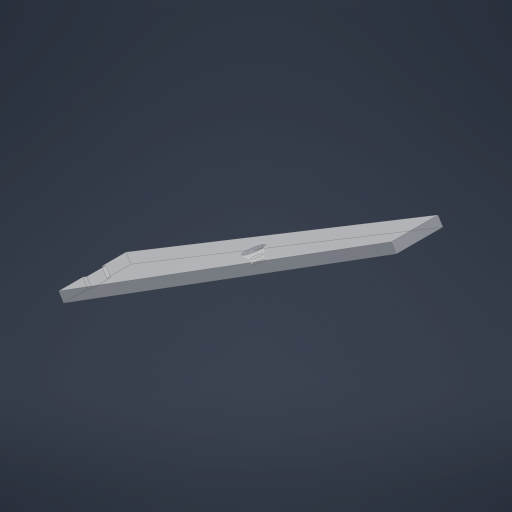
# Autodesk Inventor part: Touch Fifth
Saved by Autodesk Inventor 2023 (Build 270158000, 158)
## iProperties
Created: 2022-06-12
Part Number: Touch Fifth
Material: Polycarbonate, Clear
Document SubType Name: Modeling
Designer: FizzyApple12
Density: 1.2 g/cm^3
Appearance: Polycarbonate - Clear
Author: FizzyApple12
Autodesk Inventor part; units mm, degrees
ref_plane "XZ Plane" through (0, 0, 0) normal (0, 1, 0) x (-1, 0, 0)
sketch "Sketch1" plane through (0, 0, 0) normal (1, 0, 0) x (0, 1, 0)
  circle A0 centre (0, 0) radius 431.8 construction
  line L0 (-431.2082, -22.5987) -> (-431.2082, 22.5987)
  line L1 (-431.2082, -22.5987) -> (-386.0109, -22.5987) construction
  line L2 (-431.2082, -22.5987) -> (0, 0) construction
  line L3 (0, 0) -> (-431.2082, 22.5987) construction
  dimension "d0" = 863.6
  dimension "d3" = 90
  dimension "d4" = 6
  constraints: 8 end point, 2 point on circle, 1 centre point, 1 coincident, 1 horizontal, 1 perpendicular
  measures "d0" diameter of A0
  measures "d3" angle of L1 L0
  measures "d4" angle of L3 L2
ref_plane "Work Plane1" through (216.1794, 0, 0) normal (1, 0, 0) x (0, 1, 0)
sketch "Sketch2" plane through (216.1794, 0, 0) normal (1, 0, 0) x (0, 1, 0)
  circle A0 centre (0, 0) radius 298.45 construction
  line L0 (-298.041, 15.6197) -> (-298.041, -15.6197)
  line L1 (-298.041, 15.6197) -> (-266.8017, 15.6197) construction
  line L2 (-298.041, 15.6197) -> (0, 0) construction
  line L3 (0, 0) -> (-298.041, -15.6197) construction
  dimension "d2" = 596.9
  dimension "d5" = 90
  dimension "d6" = 6
  constraints: 8 end point, 2 point on circle, 1 centre point, 1 coincident, 1 horizontal, 1 perpendicular
  measures "d2" diameter of A0
  measures "d5" angle of L0 L1
  measures "d6" angle of L3 L2
ref_plane "Work Plane2" through (0, -431.2082, -22.5987) normal (-0.5244795, 0.8514231, 0) x (0, 0, 1)
sketch "Sketch3" plane through (0, -431.2082, -22.5987) normal (-0.5244795, 0.8514231, 0) x (0, 0, 1)
  line L0 (0, 0) -> (45.1973, 0) projected
  line L1 (38.2183, 253.9036) -> (6.979, 253.9036) projected
  line L2 (6.979, 253.9036) -> (0, 0)
  line L3 (45.1973, 0) -> (38.2183, 253.9036)
  point P0 (22.5987, 226.1599)
  constraints: 4 end point
extrude "Extrusion1" add sketch "Sketch3" against normal blind 6.35
sketch "Sketch5" plane through (0, -431.2082, -22.5987) normal (-0.5244795, 0.8514231, 0) x (0.8514231, 0.5244795, 0)
  line L0 (-3.175, -28.9487) -> (3.175, -28.9487)
  line L1 (3.175, -28.9487) -> (3.175, -16.2487)
  line L2 (3.175, -16.2487) -> (-3.175, -16.2487)
  line L3 (-3.175, -16.2487) -> (-3.175, -28.9487)
  line L4 (0, -45.1973) -> (0, 0) projected
  line L5 (-3.175, -28.9487) -> (3.175, -16.2487) construction
  line L6 (3.175, -28.9487) -> (-3.175, -16.2487) construction
  point P0 (226.1599, -22.5987)
  point P1 (0, -22.5987)
  point P2 (0, -28.9487)
  point P3 (0, -16.2487)
  dimension "d17" = 6.35
  dimension "d18" = 12.7
  constraints: 12 end point, 3 midpoint, 2 parallel, 1 horizontal, 1 perpendicular
  measures "d17" distance of L2.end L1.end
  measures "d18" distance of L1.end L0.end
extrude "Extrusion3" cut sketch "Sketch5" against normal through all
sketch "Sketch6" plane through (0, -431.2082, -22.5987) normal (-0.5244795, 0.8514231, 0) x (0.8514231, 0.5244795, 0)
  line L0 (253.9036, -38.2183) -> (253.9036, -6.979) projected
  line L1 (0, 0) -> (0, -16.2487) projected
  line L2 (253.9036, -6.979) -> (253.9036, -38.2183) projected
  line L3 (253.9036, -22.5987) -> (3.175, -22.5987) construction
  line L4 (3.175, -16.2487) -> (3.175, -28.9487) projected
  point P0 (226.1599, -22.5987)
  point P1 (126.9518, -22.5987)
  dimension "d21" = 253.9036
  dimension "d22" = 126.9518
  constraints: 2 end point, 2 midpoint, 1 point on line
  measures "d21" distance between parallel lines of L0 L1
  measures "d22" distance from line of L0 point (126.952, -22.599)
hole "Hole1" at (108.0897, -364.6246, 0) direction (0.5244795, -0.8514231, 0) diameter 6.7564 end through all countersink diameter 12.8778 countersink angle 82 clearance for "Flat Head Machine Screw (82)" size "1/4" standard "Ansi Unified Screw Threads"
equation "\"d22\" = 0.5 * d21"
body "Solid1"
